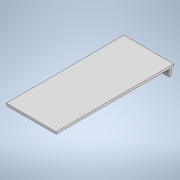
# Autodesk Inventor part: False_Bottom_2
Saved by Autodesk Inventor 2020 (Build 240168000, 168)
## iProperties
Created: 2021-12-09
Part Number: False_Bottom_2
Material: Generic
Document SubType Name: Modeling
Designer: danie
Density: 1 g/cm^3
Appearance: Default
Author: danie
Autodesk Inventor part; units mm, degrees
ref_plane "YZ Plane" through (0, 0, 0) normal (1, 0, 0) x (0, 1, 0)
ref_plane "XZ Plane" through (0, 0, 0) normal (0, 1, 0) x (-1, 0, 0)
ref_plane "XY Plane" through (0, 0, 0) normal (0, 0, 1) x (1, 0, 0)
sketch "Sketch1" plane through (0, 0, 0) normal (0, 1, 0) x (-1, 0, 0)
  line L0 (-1.4756, 0) -> (-71.3256, 0)
  line L1 (-71.3256, 0) -> (-71.3256, 165.1)
  line L2 (-71.3256, 165.1) -> (-1.4756, 165.1)
  line L3 (-1.4756, 165.1) -> (-1.4756, 0)
  point P0 (0, 0)
  dimension "d0" = 69.85
  dimension "d1" = 165.1
  constraints: 8 end point, 2 parallel, 1 horizontal, 1 perpendicular
  measures "d0" distance of L1.end L2.end
  measures "d1" distance of L0.end L1.end
extrude "Extrusion1" add sketch "Sketch1" along normal blind 3.175
sketch "Sketch3" plane through (0, 0, 0) normal (0, -1, 0) x (1, 0, 0)
  line L0 (71.3256, 165.1) -> (71.3256, 0) construction
  line L1 (71.3256, 0) -> (68.1506, 0) construction
  line L2 (71.3256, 0) -> (1.4756, 0) construction
  line L3 (1.4756, 0) -> (4.6506, 0) construction
  line L4 (68.1506, 0) -> (4.6506, 0)
  line L5 (4.6506, 0) -> (4.6506, 3.175)
  line L6 (4.6506, 3.175) -> (68.1506, 3.175)
  line L7 (68.1506, 3.175) -> (68.1506, 0)
  point P0 (0, 0)
  dimension "d7" = 3.175
  dimension "d8" = 3.175
  dimension "d9" = 63.5
  dimension "d10" = 3.175
  constraints: 12 end point, 2 parallel, 2 point on line, 1 horizontal, 1 perpendicular
  measures "d7" distance of L0.end L1.end
  measures "d8" distance of L2.end L3.end
  measures "d9" distance of L5.end L6.end
  measures "d10" distance of L4.end L5.end
extrude "Extrusion3" add sketch "Sketch3" along normal blind 12.7
body "Solid1"
